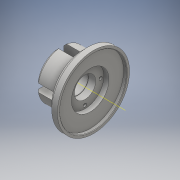
# Autodesk Inventor part: Деталь 5
Saved by Autodesk Inventor 2016 SP1 (Build 200210100, 210)
## iProperties
Created: 2016-05-02
Part Number: Деталь 5
Material: Типовые
Document SubType Name: Modeling
Designer: AS
Density: 1 g/cm^3
Appearance: По умолчанию
Author: AS
Autodesk Inventor part; units mm, degrees
ref_plane "YZ Plane" through (0, 0, 0) normal (1, 0, 0) x (0, 1, 0)
ref_plane "XZ Plane" through (0, 0, 0) normal (0, 1, 0) x (-1, 0, 0)
ref_plane "XY Plane" through (0, 0, 0) normal (0, 0, 1) x (1, 0, 0)
sketch "Эскиз1" plane through (0, 0, 0) normal (0, 0, 1) x (1, 0, 0)
  line L0 (-82.5274, -21.6687) -> (-82.5274, -51.6687)
  line L1 (-82.5274, -51.6687) -> (-32.5274, -51.6687)
  line L2 (-32.5274, -51.6687) -> (-32.5274, -76.6687)
  line L3 (-32.5274, -76.6687) -> (-10.5274, -76.6687)
  line L4 (-10.5274, -76.6687) -> (-10.5274, -71)
  line L5 (-10.5274, -71) -> (-17.5274, -71)
  line L6 (-17.5274, -71) -> (-17.5274, -40)
  line L7 (-17.5274, -40) -> (-28.5274, -40)
  line L8 (-28.5274, -40) -> (-28.5274, -22.6687)
  line L9 (-28.5274, -22.6687) -> (-43.5274, -22.6687)
  line L10 (-43.5274, -21.6687) -> (-82.5274, -21.6687)
  line L11 (-43.5274, -21.6687) -> (-43.5274, -22.6687)
  line L12 (-99.0329, 0) -> (16.5055, 0) projected
  point P0 (0, 0)
  dimension "d0" = 72
  dimension "d1" = 22
  dimension "d4" = 55
  dimension "d5" = 30
  dimension "d6" = 7
  dimension "d7" = 11
  dimension "d9" = 15
  dimension "d10" = 1
  dimension "d13" = 71
  dimension "d20" = 40
  constraints: 24 end point, 8 perpendicular, 2 vertical, 1 parallel
  measures "d0" distance between parallel lines of L0 L4
  measures "d1" distance from line of L2.end L4
  measures "d4" distance between parallel lines of L10 L3
  measures "d5" distance of L0.start L0.end
  measures "d6" distance of L5.end L4.end
  measures "d7" distance between parallel lines of L8 L6
  measures "d9" distance between parallel lines of L11 L8
  measures "d10" distance of L10.start L9.end
  measures "d13" distance between parallel lines of L5 L12
  measures "d20" distance between parallel lines of L7 L12
revolve "Вращение1" add sketch "Эскиз1" angle 360 about axis through (-10, 0, 0) along (1, 0, 0)
chamfer "Фаска1" distance 6 angle 45 1 edges at (-82.5274, 51.6687, 0)
chamfer "Фаска2" distance 10 angle 45 1 edges at (-32.5274, 76.6687, 0)
sketch "Эскиз2" plane through (-82.5274, 0, 0) normal (-1, 0, 0) x (0, 0, 1)
  arc A0 (33.1576, 8.7669) -> (33.1576, -8.2331) centre (33.1576, 0.2669) ccw
  line L0 (33.1576, -8.2331) -> (62.3415, -8.2331)
  line L1 (33.1576, 8.7669) -> (62.3415, 8.7669)
  line L2 (62.3415, 8.7669) -> (62.3415, -8.2331)
  point P0 (0, 0)
  dimension "d21" = 17
  constraints: 6 end point, 2 horizontal, 2 point on circle, 2 tangent, 1 centre point, 1 perpendicular
  measures "d21" diameter of A0
extrude "Выдавливание1" cut sketch "Эскиз2" against normal blind 50
pattern_circular "Круговой массив1" count 4 over 360 about axis through (-10, 0, 0) along (1, 0, 0) of "Выдавливание1"
hole "Отверстие1" at (-32.5274, 0.2669, 33.1576) direction (1, 0, 0) diameter 7 end through all
pattern_circular "Круговой массив2" count 4 over 360 about axis through (-10, 0, 0) along (1, 0, 0) of "Отверстие1"
fillet "Сопряжение1" radius 3 4 edges at (-32.5274, 36.3435, -36.7261) (-32.5274, 36.7261, 36.3435) (-32.5274, -36.3435, 36.7261) (-32.5274, -36.7261, -36.3435)
chamfer "Фаска3" distance 1 angle 45 1 edges at (-10.5274, 71, 0)
chamfer "Фаска4" distance 2 angle 45 1 edges at (-82.5274, 21.6687, 0)
